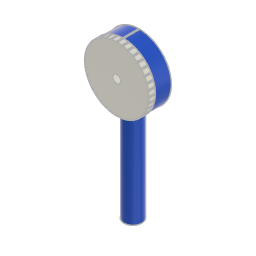
Optica-zelf-geprint (Autodesk Fusion 360 design; units mm, degrees)
Autodesk Fusion 360 part; units mm, degrees
note: some values were not read from the file. Chosen so that the rebuilt part matches the saved one: a side; which face or edge a step refers to. Set by a fixed rule: which sketch regions a step uses.
sketch "Sketch1" plane through (0, 0, 0) normal (0, 1, 0) x (1, 0, 0) in component "Bearing"
  circle A0 centre (0, 0) radius 11
  circle A1 centre (0, 0) radius 4
  dimension "d1" = 22
  dimension "d2" = 8
  constraint coincident A0.centre A1.centre
  measures "d1" diameter of A0
  measures "d2" diameter of A1
extrude "Extrude1" add sketch "Sketch1" along normal blind 7 makes body 1 in component "Bearing"
sketch "Sketch1 (2)" plane through (0, 0, 0) normal (0, -1, 0) x (1, 0, 0) in component "Rotating"
  circle A0 centre (0, 0) radius 4
  circle A1 centre (0, 0) radius 11
  circle A2 centre (0, 0) radius 3.9
  circle A3 centre (0, 0) radius 3.1
  circle A4 centre (0, 0) radius 6.5
  circle A5 centre (0, 0) radius 25
  dimension "d5" = -0.1
  dimension "d10" = -0.9
  dimension "d54" = 2.5
  dimension "d61" = 50
  constraint coincident A0.centre A1.centre
  measures "d61" diameter of A5
extrude "Extrude5" add sketch "Sketch1 (2)" along normal blind 0.5 separate body contours A0 | A4 makes body 2 in component "Rotating"
extrude "Extrude6" add sketch "Sketch1 (2)" along normal up to surface (0.5 mm away) and the other way up to surface (7 mm away) contours A2 bodies 2 in component "Rotating"
extrude "Extrude7" add sketch "Sketch1 (2)" along normal blind 5 from surface at 0.5 contours A0 | A1 | A2 | A4 | A5 bodies 2 in component "Rotating"
sketch "Sketch4" plane through (0, -5.5, 0) normal (0, -1, 0) x (1, 0, 0) in component "Rotating"
  circle A0 centre (0, 0) radius 3.1
  circle A1 centre (0, 0) radius 25
  line L0 (0, 0) -> (0, 25) construction
  line L1 (-0.5, 24.995) -> (0.5, 24.995)
  circle A2 centre (0, 0) radius 25 construction
  line L2 (-0.5, 24.995) -> (0.5, 24.995)
  line L3 (0.5, 24.995) -> (0.5, 24.195)
  line L4 (0.3, 23.995) -> (-0.3, 23.995)
  line L5 (-0.5, 24.195) -> (-0.5, 24.995)
  arc A3 (-0.5, 24.195) -> (-0.3, 23.995) centre (-0.3, 24.195) ccw
  arc A4 (0.3, 23.995) -> (0.5, 24.195) centre (0.3, 24.195) ccw
  line L6 (-3.8479, 24.7021) -> (-3.709, 23.9142)
  arc A5 (-3.8712, 23.6826) -> (-3.709, 23.9142) centre (-3.906, 23.8795) ccw
  line L7 (-3.8712, 23.6826) -> (-4.4621, 23.5784)
  arc A6 (-4.6938, 23.7406) -> (-4.4621, 23.5784) centre (-4.4969, 23.7753) ccw
  line L8 (-4.6938, 23.7406) -> (-4.8327, 24.5284)
  line L9 (-4.8327, 24.5284) -> (-3.8479, 24.7021)
  line L10 (-8.0789, 23.6586) -> (-7.8053, 22.9069)
  arc A7 (-7.9249, 22.6505) -> (-7.8053, 22.9069) centre (-7.9933, 22.8385) ccw
  line L11 (-7.9249, 22.6505) -> (-8.4887, 22.4453)
  arc A8 (-8.745, 22.5649) -> (-8.4887, 22.4453) centre (-8.5571, 22.6333) ccw
  line L12 (-8.745, 22.5649) -> (-9.0186, 23.3166)
  line L13 (-9.0186, 23.3166) -> (-8.0789, 23.6586)
  line L14 (-12.0645, 21.8963) -> (-11.6645, 21.2035)
  arc A9 (-11.7377, 20.9303) -> (-11.6645, 21.2035) centre (-11.8377, 21.1035) ccw
  line L15 (-11.7377, 20.9303) -> (-12.2573, 20.6303)
  arc A10 (-12.5305, 20.7035) -> (-12.2573, 20.6303) centre (-12.3573, 20.8035) ccw
  line L16 (-12.5305, 20.7035) -> (-12.9305, 21.3963)
  line L17 (-12.9305, 21.3963) -> (-12.0645, 21.8963)
  line L18 (-15.6835, 19.4687) -> (-15.1692, 18.8558)
  arc A11 (-15.1939, 18.5741) -> (-15.1692, 18.8558) centre (-15.3224, 18.7273) ccw
  line L19 (-15.1939, 18.5741) -> (-15.6535, 18.1884)
  arc A12 (-15.9353, 18.2131) -> (-15.6535, 18.1884) centre (-15.7821, 18.3416) ccw
  line L20 (-15.9353, 18.2131) -> (-16.4495, 18.8259)
  line L21 (-16.4495, 18.8259) -> (-15.6835, 19.4687)
  line L22 (-18.8259, 16.4495) -> (-18.2131, 15.9353)
  arc A13 (-18.1884, 15.6535) -> (-18.2131, 15.9353) centre (-18.3416, 15.7821) ccw
  line L23 (-18.1884, 15.6535) -> (-18.5741, 15.1939)
  arc A14 (-18.8558, 15.1692) -> (-18.5741, 15.1939) centre (-18.7273, 15.3224) ccw
  line L24 (-18.8558, 15.1692) -> (-19.4687, 15.6835)
  line L25 (-19.4687, 15.6835) -> (-18.8259, 16.4495)
  line L26 (-21.3963, 12.9305) -> (-20.7035, 12.5305)
  arc A15 (-20.6303, 12.2573) -> (-20.7035, 12.5305) centre (-20.8035, 12.3573) ccw
  line L27 (-20.6303, 12.2573) -> (-20.9303, 11.7377)
  arc A16 (-21.2035, 11.6645) -> (-20.9303, 11.7377) centre (-21.1035, 11.8377) ccw
  line L28 (-21.2035, 11.6645) -> (-21.8963, 12.0645)
  line L29 (-21.8963, 12.0645) -> (-21.3963, 12.9305)
  line L30 (-23.3166, 9.0186) -> (-22.5649, 8.745)
  arc A17 (-22.4453, 8.4887) -> (-22.5649, 8.745) centre (-22.6333, 8.5571) ccw
  line L31 (-22.4453, 8.4887) -> (-22.6505, 7.9249)
  arc A18 (-22.9069, 7.8053) -> (-22.6505, 7.9249) centre (-22.8385, 7.9933) ccw
  line L32 (-22.9069, 7.8053) -> (-23.6586, 8.0789)
  line L33 (-23.6586, 8.0789) -> (-23.3166, 9.0186)
  line L34 (-24.5284, 4.8327) -> (-23.7406, 4.6938)
  arc A19 (-23.5784, 4.4621) -> (-23.7406, 4.6938) centre (-23.7753, 4.4969) ccw
  line L35 (-23.5784, 4.4621) -> (-23.6826, 3.8712)
  arc A20 (-23.9142, 3.709) -> (-23.6826, 3.8712) centre (-23.8795, 3.906) ccw
  line L36 (-23.9142, 3.709) -> (-24.7021, 3.8479)
  line L37 (-24.7021, 3.8479) -> (-24.5284, 4.8327)
  line L38 (-24.995, 0.5) -> (-24.195, 0.5)
  arc A21 (-23.995, 0.3) -> (-24.195, 0.5) centre (-24.195, 0.3) ccw
  line L39 (-23.995, 0.3) -> (-23.995, -0.3)
  arc A22 (-24.195, -0.5) -> (-23.995, -0.3) centre (-24.195, -0.3) ccw
  line L40 (-24.195, -0.5) -> (-24.995, -0.5)
  line L41 (-24.995, -0.5) -> (-24.995, 0.5)
  line L42 (-24.7021, -3.8479) -> (-23.9142, -3.709)
  arc A23 (-23.6826, -3.8712) -> (-23.9142, -3.709) centre (-23.8795, -3.906) ccw
  line L43 (-23.6826, -3.8712) -> (-23.5784, -4.4621)
  arc A24 (-23.7406, -4.6938) -> (-23.5784, -4.4621) centre (-23.7753, -4.4969) ccw
  line L44 (-23.7406, -4.6938) -> (-24.5284, -4.8327)
  line L45 (-24.5284, -4.8327) -> (-24.7021, -3.8479)
  line L46 (-23.6586, -8.0789) -> (-22.9069, -7.8053)
  arc A25 (-22.6505, -7.9249) -> (-22.9069, -7.8053) centre (-22.8385, -7.9933) ccw
  line L47 (-22.6505, -7.9249) -> (-22.4453, -8.4887)
  arc A26 (-22.5649, -8.745) -> (-22.4453, -8.4887) centre (-22.6333, -8.5571) ccw
  line L48 (-22.5649, -8.745) -> (-23.3166, -9.0186)
  line L49 (-23.3166, -9.0186) -> (-23.6586, -8.0789)
  line L50 (-21.8963, -12.0645) -> (-21.2035, -11.6645)
  arc A27 (-20.9303, -11.7377) -> (-21.2035, -11.6645) centre (-21.1035, -11.8377) ccw
  line L51 (-20.9303, -11.7377) -> (-20.6303, -12.2573)
  arc A28 (-20.7035, -12.5305) -> (-20.6303, -12.2573) centre (-20.8035, -12.3573) ccw
  line L52 (-20.7035, -12.5305) -> (-21.3963, -12.9305)
  line L53 (-21.3963, -12.9305) -> (-21.8963, -12.0645)
  line L54 (-19.4687, -15.6835) -> (-18.8558, -15.1692)
  arc A29 (-18.5741, -15.1939) -> (-18.8558, -15.1692) centre (-18.7273, -15.3224) ccw
  line L55 (-18.5741, -15.1939) -> (-18.1884, -15.6535)
  arc A30 (-18.2131, -15.9353) -> (-18.1884, -15.6535) centre (-18.3416, -15.7821) ccw
  line L56 (-18.2131, -15.9353) -> (-18.8259, -16.4495)
  line L57 (-18.8259, -16.4495) -> (-19.4687, -15.6835)
  line L58 (-16.4495, -18.8259) -> (-15.9353, -18.2131)
  arc A31 (-15.6535, -18.1884) -> (-15.9353, -18.2131) centre (-15.7821, -18.3416) ccw
  line L59 (-15.6535, -18.1884) -> (-15.1939, -18.5741)
  arc A32 (-15.1692, -18.8558) -> (-15.1939, -18.5741) centre (-15.3224, -18.7273) ccw
  line L60 (-15.1692, -18.8558) -> (-15.6835, -19.4687)
  line L61 (-15.6835, -19.4687) -> (-16.4495, -18.8259)
  line L62 (-12.9305, -21.3963) -> (-12.5305, -20.7035)
  arc A33 (-12.2573, -20.6303) -> (-12.5305, -20.7035) centre (-12.3573, -20.8035) ccw
  line L63 (-12.2573, -20.6303) -> (-11.7377, -20.9303)
  arc A34 (-11.6645, -21.2035) -> (-11.7377, -20.9303) centre (-11.8377, -21.1035) ccw
  line L64 (-11.6645, -21.2035) -> (-12.0645, -21.8963)
  line L65 (-12.0645, -21.8963) -> (-12.9305, -21.3963)
  line L66 (-9.0186, -23.3166) -> (-8.745, -22.5649)
  arc A35 (-8.4887, -22.4453) -> (-8.745, -22.5649) centre (-8.5571, -22.6333) ccw
  line L67 (-8.4887, -22.4453) -> (-7.9249, -22.6505)
  arc A36 (-7.8053, -22.9069) -> (-7.9249, -22.6505) centre (-7.9933, -22.8385) ccw
  line L68 (-7.8053, -22.9069) -> (-8.0789, -23.6586)
  line L69 (-8.0789, -23.6586) -> (-9.0186, -23.3166)
  line L70 (-4.8327, -24.5284) -> (-4.6938, -23.7406)
  arc A37 (-4.4621, -23.5784) -> (-4.6938, -23.7406) centre (-4.4969, -23.7753) ccw
  line L71 (-4.4621, -23.5784) -> (-3.8712, -23.6826)
  arc A38 (-3.709, -23.9142) -> (-3.8712, -23.6826) centre (-3.906, -23.8795) ccw
  line L72 (-3.709, -23.9142) -> (-3.8479, -24.7021)
  line L73 (-3.8479, -24.7021) -> (-4.8327, -24.5284)
  line L74 (-0.5, -24.995) -> (-0.5, -24.195)
  arc A39 (-0.3, -23.995) -> (-0.5, -24.195) centre (-0.3, -24.195) ccw
  line L75 (-0.3, -23.995) -> (0.3, -23.995)
  arc A40 (0.5, -24.195) -> (0.3, -23.995) centre (0.3, -24.195) ccw
  line L76 (0.5, -24.195) -> (0.5, -24.995)
  line L77 (0.5, -24.995) -> (-0.5, -24.995)
  line L78 (3.8479, -24.7021) -> (3.709, -23.9142)
  arc A41 (3.8712, -23.6826) -> (3.709, -23.9142) centre (3.906, -23.8795) ccw
  line L79 (3.8712, -23.6826) -> (4.4621, -23.5784)
  arc A42 (4.6938, -23.7406) -> (4.4621, -23.5784) centre (4.4969, -23.7753) ccw
  line L80 (4.6938, -23.7406) -> (4.8327, -24.5284)
  line L81 (4.8327, -24.5284) -> (3.8479, -24.7021)
  line L82 (8.0789, -23.6586) -> (7.8053, -22.9069)
  arc A43 (7.9249, -22.6505) -> (7.8053, -22.9069) centre (7.9933, -22.8385) ccw
  line L83 (7.9249, -22.6505) -> (8.4887, -22.4453)
  arc A44 (8.745, -22.5649) -> (8.4887, -22.4453) centre (8.5571, -22.6333) ccw
  line L84 (8.745, -22.5649) -> (9.0186, -23.3166)
  line L85 (9.0186, -23.3166) -> (8.0789, -23.6586)
  line L86 (12.0645, -21.8963) -> (11.6645, -21.2035)
  arc A45 (11.7377, -20.9303) -> (11.6645, -21.2035) centre (11.8377, -21.1035) ccw
  line L87 (11.7377, -20.9303) -> (12.2573, -20.6303)
  arc A46 (12.5305, -20.7035) -> (12.2573, -20.6303) centre (12.3573, -20.8035) ccw
  line L88 (12.5305, -20.7035) -> (12.9305, -21.3963)
  line L89 (12.9305, -21.3963) -> (12.0645, -21.8963)
  line L90 (15.6835, -19.4687) -> (15.1692, -18.8558)
  arc A47 (15.1939, -18.5741) -> (15.1692, -18.8558) centre (15.3224, -18.7273) ccw
  line L91 (15.1939, -18.5741) -> (15.6535, -18.1884)
  arc A48 (15.9353, -18.2131) -> (15.6535, -18.1884) centre (15.7821, -18.3416) ccw
  line L92 (15.9353, -18.2131) -> (16.4495, -18.8259)
  line L93 (16.4495, -18.8259) -> (15.6835, -19.4687)
  line L94 (18.8259, -16.4495) -> (18.2131, -15.9353)
  arc A49 (18.1884, -15.6535) -> (18.2131, -15.9353) centre (18.3416, -15.7821) ccw
  line L95 (18.1884, -15.6535) -> (18.5741, -15.1939)
  arc A50 (18.8558, -15.1692) -> (18.5741, -15.1939) centre (18.7273, -15.3224) ccw
  line L96 (18.8558, -15.1692) -> (19.4687, -15.6835)
  line L97 (19.4687, -15.6835) -> (18.8259, -16.4495)
  line L98 (21.3963, -12.9305) -> (20.7035, -12.5305)
  arc A51 (20.6303, -12.2573) -> (20.7035, -12.5305) centre (20.8035, -12.3573) ccw
  line L99 (20.6303, -12.2573) -> (20.9303, -11.7377)
  arc A52 (21.2035, -11.6645) -> (20.9303, -11.7377) centre (21.1035, -11.8377) ccw
  line L100 (21.2035, -11.6645) -> (21.8963, -12.0645)
  line L101 (21.8963, -12.0645) -> (21.3963, -12.9305)
  line L102 (23.3166, -9.0186) -> (22.5649, -8.745)
  arc A53 (22.4453, -8.4887) -> (22.5649, -8.745) centre (22.6333, -8.5571) ccw
  line L103 (22.4453, -8.4887) -> (22.6505, -7.9249)
  arc A54 (22.9069, -7.8053) -> (22.6505, -7.9249) centre (22.8385, -7.9933) ccw
  line L104 (22.9069, -7.8053) -> (23.6586, -8.0789)
  line L105 (23.6586, -8.0789) -> (23.3166, -9.0186)
  line L106 (24.5284, -4.8327) -> (23.7406, -4.6938)
  arc A55 (23.5784, -4.4621) -> (23.7406, -4.6938) centre (23.7753, -4.4969) ccw
  line L107 (23.5784, -4.4621) -> (23.6826, -3.8712)
  arc A56 (23.9142, -3.709) -> (23.6826, -3.8712) centre (23.8795, -3.906) ccw
  line L108 (23.9142, -3.709) -> (24.7021, -3.8479)
  line L109 (24.7021, -3.8479) -> (24.5284, -4.8327)
  line L110 (24.995, -0.5) -> (24.195, -0.5)
  arc A57 (23.995, -0.3) -> (24.195, -0.5) centre (24.195, -0.3) ccw
  line L111 (23.995, -0.3) -> (23.995, 0.3)
  arc A58 (24.195, 0.5) -> (23.995, 0.3) centre (24.195, 0.3) ccw
  line L112 (24.195, 0.5) -> (24.995, 0.5)
  line L113 (24.995, 0.5) -> (24.995, -0.5)
  line L114 (24.7021, 3.8479) -> (23.9142, 3.709)
  arc A59 (23.6826, 3.8712) -> (23.9142, 3.709) centre (23.8795, 3.906) ccw
  line L115 (23.6826, 3.8712) -> (23.5784, 4.4621)
  arc A60 (23.7406, 4.6938) -> (23.5784, 4.4621) centre (23.7753, 4.4969) ccw
  line L116 (23.7406, 4.6938) -> (24.5284, 4.8327)
  line L117 (24.5284, 4.8327) -> (24.7021, 3.8479)
  line L118 (23.6586, 8.0789) -> (22.9069, 7.8053)
  arc A61 (22.6505, 7.9249) -> (22.9069, 7.8053) centre (22.8385, 7.9933) ccw
  line L119 (22.6505, 7.9249) -> (22.4453, 8.4887)
  arc A62 (22.5649, 8.745) -> (22.4453, 8.4887) centre (22.6333, 8.5571) ccw
  line L120 (22.5649, 8.745) -> (23.3166, 9.0186)
  line L121 (23.3166, 9.0186) -> (23.6586, 8.0789)
  line L122 (21.8963, 12.0645) -> (21.2035, 11.6645)
  arc A63 (20.9303, 11.7377) -> (21.2035, 11.6645) centre (21.1035, 11.8377) ccw
  line L123 (20.9303, 11.7377) -> (20.6303, 12.2573)
  arc A64 (20.7035, 12.5305) -> (20.6303, 12.2573) centre (20.8035, 12.3573) ccw
  line L124 (20.7035, 12.5305) -> (21.3963, 12.9305)
  line L125 (21.3963, 12.9305) -> (21.8963, 12.0645)
  line L126 (19.4687, 15.6835) -> (18.8558, 15.1692)
  arc A65 (18.5741, 15.1939) -> (18.8558, 15.1692) centre (18.7273, 15.3224) ccw
  line L127 (18.5741, 15.1939) -> (18.1884, 15.6535)
  arc A66 (18.2131, 15.9353) -> (18.1884, 15.6535) centre (18.3416, 15.7821) ccw
  line L128 (18.2131, 15.9353) -> (18.8259, 16.4495)
  line L129 (18.8259, 16.4495) -> (19.4687, 15.6835)
  line L130 (16.4495, 18.8259) -> (15.9353, 18.2131)
  arc A67 (15.6535, 18.1884) -> (15.9353, 18.2131) centre (15.7821, 18.3416) ccw
  line L131 (15.6535, 18.1884) -> (15.1939, 18.5741)
  arc A68 (15.1692, 18.8558) -> (15.1939, 18.5741) centre (15.3224, 18.7273) ccw
  line L132 (15.1692, 18.8558) -> (15.6835, 19.4687)
  line L133 (15.6835, 19.4687) -> (16.4495, 18.8259)
  line L134 (12.9305, 21.3963) -> (12.5305, 20.7035)
  arc A69 (12.2573, 20.6303) -> (12.5305, 20.7035) centre (12.3573, 20.8035) ccw
  line L135 (12.2573, 20.6303) -> (11.7377, 20.9303)
  arc A70 (11.6645, 21.2035) -> (11.7377, 20.9303) centre (11.8377, 21.1035) ccw
  line L136 (11.6645, 21.2035) -> (12.0645, 21.8963)
  line L137 (12.0645, 21.8963) -> (12.9305, 21.3963)
  line L138 (9.0186, 23.3166) -> (8.745, 22.5649)
  arc A71 (8.4887, 22.4453) -> (8.745, 22.5649) centre (8.5571, 22.6333) ccw
  line L139 (8.4887, 22.4453) -> (7.9249, 22.6505)
  arc A72 (7.8053, 22.9069) -> (7.9249, 22.6505) centre (7.9933, 22.8385) ccw
  line L140 (7.8053, 22.9069) -> (8.0789, 23.6586)
  line L141 (8.0789, 23.6586) -> (9.0186, 23.3166)
  line L142 (4.8327, 24.5284) -> (4.6938, 23.7406)
  arc A73 (4.4621, 23.5784) -> (4.6938, 23.7406) centre (4.4969, 23.7753) ccw
  line L143 (4.4621, 23.5784) -> (3.8712, 23.6826)
  arc A74 (3.709, 23.9142) -> (3.8712, 23.6826) centre (3.906, 23.8795) ccw
  line L144 (3.709, 23.9142) -> (3.8479, 24.7021)
  line L145 (3.8479, 24.7021) -> (4.8327, 24.5284)
  line L146 (-4.7516, 24.6443) -> (-3.9638, 24.7832)
  line L147 (-3.8479, 24.7021) -> (-4.8327, 24.5284)
  arc A75 (-4.7516, 24.6443) -> (-4.8327, 24.5284) centre (-4.7343, 24.5458) ccw
  arc A76 (-3.8479, 24.7021) -> (-3.9638, 24.7832) centre (-3.9464, 24.6847) ccw
  point P0 (0, 24.995)
  point P1 (-0.5, 23.995)
  dimension "d65" = 1
  dimension "d70" = 1
  dimension "d71" = 0.2
  dimension "d73" = 360
  dimension "d76" = 0.1
  dimension "d77" = 0.1
  dimension "d78" = 0.8
  constraint coincident A0.centre A1.centre
  constraint coincident A1 L0.end
  constraint vertical L0
  constraint perpendicular L0 L1
  constraint midpoint L1 P0
  constraint coincident L0 P0
  constraint coincident L1.start A2
  constraint perpendicular L2 L3
  constraint parallel L2 L4
  constraint parallel L3 L5
  constraint coincident P1 L4
  constraint coincident P1 L5
  constraint tangent L4 A3
  constraint tangent L5 A3
  constraint tangent L3 A4
  constraint tangent L4 A4
  constraint equal A3 A4
  constraint parallel L146 L147
  constraint tangent L146 A75
  constraint coincident L8.end L9.start
  constraint tangent L146 A76
  constraint equal A75 A76
  constraint coincident L6.start L9.end
  measures "d65" distance of L1.start L1.end
  measures "d70" distance of L1.start P1
  measures "d71" radius of A3
  measures "d76" radius of A75
  measures "d77" distance of L146 L147
  measures "d78" distance of L146.start L146.end
extrude "Extrude8" add sketch "Sketch4" against normal blind 5 contours A1 L146 A75 A76 bodies 2 in component "Rotating"
pattern_circular "C-Pattern1" count 36 over 360 about axis through (0, 1.75, 0) along (0, 1, 0) of "Extrude8" in component "Rotating"
extrude "Extrude9" cut sketch "Sketch4" against normal blind 0.001 contours L110 A57 L111 A58 L112 L113 | L114 A59 L115 A60 L116 L117 | L106 A55 L107 A56 L108 L109 | L118 A61 L119 A62 L120 L121 | L102 A53 L103 A54 L104 L105 | L122 A63 L123 A64 L124 L125 | L98 A51 L99 A52 L100 L101 | L126 A65 L127 A66 L128 L129 | L94 A49 L95 A50 L96 L97 | L130 A67 L131 A68 L132 L133 | L90 A47 L91 A48 L92 L93 | L134 A69 L135 A70 L136 L137 | L86 A45 L87 A46 L88 L89 | L138 A71 L139 A72 L140 L141 | L82 A43 L83 A44 L84 L85 | L142 A73 L143 A74 L144 L145 | L78 A41 L79 A42 L80 L81 | L1 L2 L3 L4 L5 A3 A4 | L74 A39 L75 A40 L76 L77 | L6 A5 L7 A6 L8 L9 L147 | L70 A37 L71 A38 L72 L73 | L10 A7 L11 A8 L12 L13 | L66 A35 L67 A36 L68 L69 | L14 A9 L15 A10 L16 L17 | L62 A33 L63 A34 L64 L65 | L18 A11 L19 A12 L20 L21 | L58 A31 L59 A32 L60 L61 | L22 A13 L23 A14 L24 L25 | L54 A29 L55 A30 L56 L57 | L26 A15 L27 A16 L28 L29 | L50 A27 L51 A28 L52 L53 | L30 A17 L31 A18 L32 L33 | L46 A25 L47 A26 L48 L49 | L34 A19 L35 A20 L36 L37 | L42 A23 L43 A24 L44 L45 | L38 A21 L39 A22 L40 L41 bodies 2 in component "Rotating"
sketch "Sketch1 (3)" plane through (0, 7, 0) normal (0, 1, 0) x (-1, 0, 0) in component "Static"
  circle A0 centre (0, 0) radius 4
  circle A1 centre (0, 0) radius 11
  circle A2 centre (0, 0) radius 3.1
  circle A3 centre (0, 0) radius 3.9
  arc A4 (3.8479, 24.7021) -> (0.5, 24.995) centre (0, 0) ccw
  arc A5 (0.5, 24.995) -> (0.4, 25.095) centre (0.4, 24.995) ccw
  line L0 (0.4, 25.095) -> (-0.4, 25.095)
  arc A6 (-0.4, 25.095) -> (-0.5, 24.995) centre (-0.4, 24.995) ccw
  arc A7 (-0.5, 24.995) -> (-3.8479, 24.7021) centre (0, 0) ccw
  arc A8 (-3.8479, 24.7021) -> (-3.9638, 24.7832) centre (-3.9464, 24.6847) ccw
  line L1 (-3.9638, 24.7832) -> (-4.7516, 24.6443)
  arc A9 (-4.7516, 24.6443) -> (-4.8327, 24.5284) centre (-4.7343, 24.5458) ccw
  arc A10 (-4.8327, 24.5284) -> (-8.0789, 23.6586) centre (0, 0) ccw
  arc A11 (-8.0789, 23.6586) -> (-8.2071, 23.7184) centre (-8.1729, 23.6244) ccw
  line L2 (-8.2071, 23.7184) -> (-8.9589, 23.4448)
  arc A12 (-8.9589, 23.4448) -> (-9.0186, 23.3166) centre (-8.9247, 23.3508) ccw
  arc A13 (-9.0186, 23.3166) -> (-12.0645, 21.8963) centre (0, 0) ccw
  arc A14 (-12.0645, 21.8963) -> (-12.2011, 21.9329) centre (-12.1511, 21.8463) ccw
  line L3 (-12.2011, 21.9329) -> (-12.8939, 21.5329)
  arc A15 (-12.8939, 21.5329) -> (-12.9305, 21.3963) centre (-12.8439, 21.4463) ccw
  arc A16 (-12.9305, 21.3963) -> (-15.6835, 19.4687) centre (0, 0) ccw
  arc A17 (-15.6835, 19.4687) -> (-15.8243, 19.481) centre (-15.7601, 19.4044) ccw
  line L4 (-15.8243, 19.481) -> (-16.4372, 18.9668)
  arc A18 (-16.4372, 18.9668) -> (-16.4495, 18.8259) centre (-16.3729, 18.8902) ccw
  arc A19 (-16.4495, 18.8259) -> (-18.8259, 16.4495) centre (0, 0) ccw
  arc A20 (-18.8259, 16.4495) -> (-18.9668, 16.4372) centre (-18.8902, 16.3729) ccw
  line L5 (-18.9668, 16.4372) -> (-19.481, 15.8243)
  arc A21 (-19.481, 15.8243) -> (-19.4687, 15.6835) centre (-19.4044, 15.7601) ccw
  arc A22 (-19.4687, 15.6835) -> (-21.3963, 12.9305) centre (0, 0) ccw
  arc A23 (-21.3963, 12.9305) -> (-21.5329, 12.8939) centre (-21.4463, 12.8439) ccw
  line L6 (-21.5329, 12.8939) -> (-21.9329, 12.2011)
  arc A24 (-21.9329, 12.2011) -> (-21.8963, 12.0645) centre (-21.8463, 12.1511) ccw
  arc A25 (-21.8963, 12.0645) -> (-23.3166, 9.0186) centre (0, 0) ccw
  arc A26 (-23.3166, 9.0186) -> (-23.4448, 8.9589) centre (-23.3508, 8.9247) ccw
  line L7 (-23.4448, 8.9589) -> (-23.7184, 8.2071)
  arc A27 (-23.7184, 8.2071) -> (-23.6586, 8.0789) centre (-23.6244, 8.1729) ccw
  arc A28 (-23.6586, 8.0789) -> (-24.5284, 4.8327) centre (0, 0) ccw
  arc A29 (-24.5284, 4.8327) -> (-24.6443, 4.7516) centre (-24.5458, 4.7343) ccw
  line L8 (-24.6443, 4.7516) -> (-24.7832, 3.9638)
  arc A30 (-24.7832, 3.9638) -> (-24.7021, 3.8479) centre (-24.6847, 3.9464) ccw
  arc A31 (-24.7021, 3.8479) -> (-24.995, 0.5) centre (0, 0) ccw
  arc A32 (-24.995, 0.5) -> (-25.095, 0.4) centre (-24.995, 0.4) ccw
  line L9 (-25.095, 0.4) -> (-25.095, -0.4)
  arc A33 (-25.095, -0.4) -> (-24.995, -0.5) centre (-24.995, -0.4) ccw
  arc A34 (-24.995, -0.5) -> (-24.7021, -3.8479) centre (0, 0) ccw
  arc A35 (-24.7021, -3.8479) -> (-24.7832, -3.9638) centre (-24.6847, -3.9464) ccw
  line L10 (-24.7832, -3.9638) -> (-24.6443, -4.7516)
  arc A36 (-24.6443, -4.7516) -> (-24.5284, -4.8327) centre (-24.5458, -4.7343) ccw
  arc A37 (-24.5284, -4.8327) -> (-23.6586, -8.0789) centre (0, 0) ccw
  arc A38 (-23.6586, -8.0789) -> (-23.7184, -8.2071) centre (-23.6244, -8.1729) ccw
  line L11 (-23.7184, -8.2071) -> (-23.4448, -8.9589)
  arc A39 (-23.4448, -8.9589) -> (-23.3166, -9.0186) centre (-23.3508, -8.9247) ccw
  arc A40 (-23.3166, -9.0186) -> (-21.8963, -12.0645) centre (0, 0) ccw
  arc A41 (-21.8963, -12.0645) -> (-21.9329, -12.2011) centre (-21.8463, -12.1511) ccw
  line L12 (-21.9329, -12.2011) -> (-21.5329, -12.8939)
  arc A42 (-21.5329, -12.8939) -> (-21.3963, -12.9305) centre (-21.4463, -12.8439) ccw
  arc A43 (-21.3963, -12.9305) -> (-19.4687, -15.6835) centre (0, 0) ccw
  arc A44 (-19.4687, -15.6835) -> (-19.481, -15.8243) centre (-19.4044, -15.7601) ccw
  line L13 (-19.481, -15.8243) -> (-18.9668, -16.4372)
  arc A45 (-18.9668, -16.4372) -> (-18.8259, -16.4495) centre (-18.8902, -16.3729) ccw
  arc A46 (-18.8259, -16.4495) -> (-16.4495, -18.8259) centre (0, 0) ccw
  arc A47 (-16.4495, -18.8259) -> (-16.4372, -18.9668) centre (-16.3729, -18.8902) ccw
  line L14 (-16.4372, -18.9668) -> (-15.8243, -19.481)
  arc A48 (-15.8243, -19.481) -> (-15.6835, -19.4687) centre (-15.7601, -19.4044) ccw
  arc A49 (-15.6835, -19.4687) -> (-12.9305, -21.3963) centre (0, 0) ccw
  arc A50 (-12.9305, -21.3963) -> (-12.8939, -21.5329) centre (-12.8439, -21.4463) ccw
  line L15 (-12.8939, -21.5329) -> (-12.2011, -21.9329)
  arc A51 (-12.2011, -21.9329) -> (-12.0645, -21.8963) centre (-12.1511, -21.8463) ccw
  arc A52 (-12.0645, -21.8963) -> (-9.0186, -23.3166) centre (0, 0) ccw
  arc A53 (-9.0186, -23.3166) -> (-8.9589, -23.4448) centre (-8.9247, -23.3508) ccw
  line L16 (-8.9589, -23.4448) -> (-8.2071, -23.7184)
  arc A54 (-8.2071, -23.7184) -> (-8.0789, -23.6586) centre (-8.1729, -23.6244) ccw
  arc A55 (-8.0789, -23.6586) -> (-4.8327, -24.5284) centre (0, 0) ccw
  arc A56 (-4.8327, -24.5284) -> (-4.7516, -24.6443) centre (-4.7343, -24.5458) ccw
  line L17 (-4.7516, -24.6443) -> (-3.9638, -24.7832)
  arc A57 (-3.9638, -24.7832) -> (-3.8479, -24.7021) centre (-3.9464, -24.6847) ccw
  arc A58 (-3.8479, -24.7021) -> (-0.5, -24.995) centre (0, 0) ccw
  arc A59 (-0.5, -24.995) -> (-0.4, -25.095) centre (-0.4, -24.995) ccw
  line L18 (-0.4, -25.095) -> (0.4, -25.095)
  arc A60 (0.4, -25.095) -> (0.5, -24.995) centre (0.4, -24.995) ccw
  arc A61 (0.5, -24.995) -> (3.8479, -24.7021) centre (0, 0) ccw
  arc A62 (3.8479, -24.7021) -> (3.9638, -24.7832) centre (3.9464, -24.6847) ccw
  line L19 (3.9638, -24.7832) -> (4.7516, -24.6443)
  arc A63 (4.7516, -24.6443) -> (4.8327, -24.5284) centre (4.7343, -24.5458) ccw
  arc A64 (4.8327, -24.5284) -> (8.0789, -23.6586) centre (0, 0) ccw
  arc A65 (8.0789, -23.6586) -> (8.2071, -23.7184) centre (8.1729, -23.6244) ccw
  line L20 (8.2071, -23.7184) -> (8.9589, -23.4448)
  arc A66 (8.9589, -23.4448) -> (9.0186, -23.3166) centre (8.9247, -23.3508) ccw
  arc A67 (9.0186, -23.3166) -> (12.0645, -21.8963) centre (0, 0) ccw
  arc A68 (12.0645, -21.8963) -> (12.2011, -21.9329) centre (12.1511, -21.8463) ccw
  line L21 (12.2011, -21.9329) -> (12.8939, -21.5329)
  arc A69 (12.8939, -21.5329) -> (12.9305, -21.3963) centre (12.8439, -21.4463) ccw
  arc A70 (12.9305, -21.3963) -> (15.6835, -19.4687) centre (0, 0) ccw
  arc A71 (15.6835, -19.4687) -> (15.8243, -19.481) centre (15.7601, -19.4044) ccw
  line L22 (15.8243, -19.481) -> (16.4372, -18.9668)
  arc A72 (16.4372, -18.9668) -> (16.4495, -18.8259) centre (16.3729, -18.8902) ccw
  arc A73 (16.4495, -18.8259) -> (18.8259, -16.4495) centre (0, 0) ccw
  arc A74 (18.8259, -16.4495) -> (18.9668, -16.4372) centre (18.8902, -16.3729) ccw
  line L23 (18.9668, -16.4372) -> (19.481, -15.8243)
  arc A75 (19.481, -15.8243) -> (19.4687, -15.6835) centre (19.4044, -15.7601) ccw
  arc A76 (19.4687, -15.6835) -> (21.3963, -12.9305) centre (0, 0) ccw
  arc A77 (21.3963, -12.9305) -> (21.5329, -12.8939) centre (21.4463, -12.8439) ccw
  line L24 (21.5329, -12.8939) -> (21.9329, -12.2011)
  arc A78 (21.9329, -12.2011) -> (21.8963, -12.0645) centre (21.8463, -12.1511) ccw
  arc A79 (21.8963, -12.0645) -> (23.3166, -9.0186) centre (0, 0) ccw
  arc A80 (23.3166, -9.0186) -> (23.4448, -8.9589) centre (23.3508, -8.9247) ccw
  line L25 (23.4448, -8.9589) -> (23.7184, -8.2071)
  arc A81 (23.7184, -8.2071) -> (23.6586, -8.0789) centre (23.6244, -8.1729) ccw
  arc A82 (23.6586, -8.0789) -> (24.5284, -4.8327) centre (0, 0) ccw
  arc A83 (24.5284, -4.8327) -> (24.6443, -4.7516) centre (24.5458, -4.7343) ccw
  line L26 (24.6443, -4.7516) -> (24.7832, -3.9638)
  arc A84 (24.7832, -3.9638) -> (24.7021, -3.8479) centre (24.6847, -3.9464) ccw
  arc A85 (24.7021, -3.8479) -> (24.995, -0.5) centre (0, 0) ccw
  arc A86 (24.995, -0.5) -> (25.095, -0.4) centre (24.995, -0.4) ccw
  line L27 (25.095, -0.4) -> (25.095, 0.4)
  arc A87 (25.095, 0.4) -> (24.995, 0.5) centre (24.995, 0.4) ccw
  arc A88 (24.995, 0.5) -> (24.7021, 3.8479) centre (0, 0) ccw
  arc A89 (24.7021, 3.8479) -> (24.7832, 3.9638) centre (24.6847, 3.9464) ccw
  line L28 (24.7832, 3.9638) -> (24.6443, 4.7516)
  arc A90 (24.6443, 4.7516) -> (24.5284, 4.8327) centre (24.5458, 4.7343) ccw
  arc A91 (24.5284, 4.8327) -> (23.6586, 8.0789) centre (0, 0) ccw
  arc A92 (23.6586, 8.0789) -> (23.7184, 8.2071) centre (23.6244, 8.1729) ccw
  line L29 (23.7184, 8.2071) -> (23.4448, 8.9589)
  arc A93 (23.4448, 8.9589) -> (23.3166, 9.0186) centre (23.3508, 8.9247) ccw
  arc A94 (23.3166, 9.0186) -> (21.8963, 12.0645) centre (0, 0) ccw
  arc A95 (21.8963, 12.0645) -> (21.9329, 12.2011) centre (21.8463, 12.1511) ccw
  line L30 (21.9329, 12.2011) -> (21.5329, 12.8939)
  arc A96 (21.5329, 12.8939) -> (21.3963, 12.9305) centre (21.4463, 12.8439) ccw
  arc A97 (21.3963, 12.9305) -> (19.4687, 15.6835) centre (0, 0) ccw
  arc A98 (19.4687, 15.6835) -> (19.481, 15.8243) centre (19.4044, 15.7601) ccw
  line L31 (19.481, 15.8243) -> (18.9668, 16.4372)
  arc A99 (18.9668, 16.4372) -> (18.8259, 16.4495) centre (18.8902, 16.3729) ccw
  arc A100 (18.8259, 16.4495) -> (16.4495, 18.8259) centre (0, 0) ccw
  arc A101 (16.4495, 18.8259) -> (16.4372, 18.9668) centre (16.3729, 18.8902) ccw
  line L32 (16.4372, 18.9668) -> (15.8243, 19.481)
  arc A102 (15.8243, 19.481) -> (15.6835, 19.4687) centre (15.7601, 19.4044) ccw
  arc A103 (15.6835, 19.4687) -> (12.9305, 21.3963) centre (0, 0) ccw
  arc A104 (12.9305, 21.3963) -> (12.8939, 21.5329) centre (12.8439, 21.4463) ccw
  line L33 (12.8939, 21.5329) -> (12.2011, 21.9329)
  arc A105 (12.2011, 21.9329) -> (12.0645, 21.8963) centre (12.1511, 21.8463) ccw
  arc A106 (12.0645, 21.8963) -> (9.0186, 23.3166) centre (0, 0) ccw
  arc A107 (9.0186, 23.3166) -> (8.9589, 23.4448) centre (8.9247, 23.3508) ccw
  line L34 (8.9589, 23.4448) -> (8.2071, 23.7184)
  arc A108 (8.2071, 23.7184) -> (8.0789, 23.6586) centre (8.1729, 23.6244) ccw
  arc A109 (8.0789, 23.6586) -> (4.8327, 24.5284) centre (0, 0) ccw
  arc A110 (4.8327, 24.5284) -> (4.7516, 24.6443) centre (4.7343, 24.5458) ccw
  line L35 (4.7516, 24.6443) -> (3.9638, 24.7832)
  arc A111 (3.9638, 24.7832) -> (3.8479, 24.7021) centre (3.9464, 24.6847) ccw
  circle A112 centre (0, 0) radius 6.5
  circle A113 centre (0, 0) radius 11.1
  circle A114 centre (0, 0) radius 25
  dimension "d79" = 0.1
  dimension "d80" = 50
  constraint concentric A4 A114
  measures "d80" diameter of A114
extrude "Extrude1'" add sketch "Sketch1 (3)" against normal up to surface (12.4 mm away) from surface at 5 separate body contours A4 A7 A10 A13 A16 A19 A22 A25 A28 A31 A34 A37 A40 A43 A46 A49 A52 A55 A58 A61 A64 A67 A70 A73 A76 A79 A82 A85 A88 A91 A94 A97 A100 A103 A106 A109 A114 | A5 L0 A6 A114 | A86 L27 A87 A114 makes body 3 in component "Static"
sketch "Sketch6" plane through (0, 12, 0) normal (0, 1, 0) x (-1, 0, 0) in component "Static"
  circle A0 centre (0, 0) radius 11.1
  arc A1 (25.095, 0.4) -> (24.995, 0.5) centre (24.995, 0.4) ccw
  arc A2 (24.995, 0.5) -> (0.5, 24.995) centre (0, 0) ccw
  arc A3 (0.5, 24.995) -> (0.4, 25.095) centre (0.4, 24.995) ccw
  line L0 (0.4, 25.095) -> (-0.4, 25.095)
  arc A4 (-0.4, 25.095) -> (-0.5, 24.995) centre (-0.4, 24.995) ccw
  arc A5 (-0.5, 24.995) -> (24.995, -0.5) centre (0, 0) ccw
  arc A6 (24.995, -0.5) -> (25.095, -0.4) centre (24.995, -0.4) ccw
  line L1 (25.095, -0.4) -> (25.095, 0.4)
  circle A7 centre (0, 0) radius 4
extrude "Extrude3" add sketch "Sketch6" against normal up to surface (4.5 mm away) contours A0 bodies 3 in component "Static"
sketch "Sketch7" plane through (0, 7.5, 0) normal (0, -1, 0) x (1, 0, 0) in component "Static"
  circle A0 centre (0, 0) radius 4
  circle A1 centre (0, 0) radius 11.1
  circle A2 centre (0, 0) radius 11.1
  circle A3 centre (0, 0) radius 9.1
  dimension "d98" = -2
extrude "Extrude4" add sketch "Sketch7" along normal up to surface (0.5 mm away) contours A1 A2 bodies 3 in component "Static"
ref_plane "WorkPlane1" through (0, 0, -25) normal (0, 0, 1) x (1, 0, 0) in component "Static"
sketch "Sketch8" plane through (0, 0, -25) normal (0, 0, 1) x (1, 0, 0) in component "Static"
  circle A0 centre (0.0267, 7) radius 7
  line L0 (11, 0) -> (-11, 0)
  line L1 (25, 12) -> (-24.995, 12)
  dimension "d102" = 14
  constraint tangent A0 L0
  measures "d102" diameter of A0
extrude "Extrude5'" add sketch "Sketch8" against normal blind 75 separate body contours A0 L1 picked at (1.7607, 8.3394) makes body 4 in component "Static"
ref_plane "WorkPlane3" through (0.0267, 6, -15) normal (0, 0, 1) x (1, 0, 0) in component "Static"
sketch "Sketch9" plane through (0, 0, -15) normal (0, 0, 1) x (1, 0, 0) in component "Static"
  line L0 (-4, 12) -> (4, 12)
  line L1 (-24.995, -0.4) -> (25, -0.4)
  line L2 (-24.995, -0.4) -> (-24.995, 12)
  line L3 (25, 12) -> (-24.995, 12)
  line L4 (-20, -0.4) -> (20, -0.4)
  line L5 (20, -0.4) -> (20, 12)
  line L6 (20, 12) -> (-20, 12)
  line L7 (-20, 12) -> (-20, -0.4)
  line L8 (-20, -0.4) -> (20, 12) construction
  line L9 (20, -0.4) -> (-20, 12) construction
  line L10 (0, 1.75) -> (0, 22.5)
  point P0 (0, 5.8)
  dimension "d106" = 40
  constraint horizontal L4
  constraint perpendicular L4 L5
  constraint parallel L4 L6
  constraint parallel L5 L7
  constraint coincident L8 P0
  constraint coincident L9 P0
  constraint coincident L1 L4.start
  constraint coincident L3 L6.end
  constraint coincident P0 L10
  measures "d106" distance of L5 L7
loft "Loft2" add profiles "Sketch9" section 1 face at (1.7607, 8.3394, -25) section 2 contours L0 L1 L3 L4 L5 L6 L7 on bodies 4 bodies 3 4 in component "Static"
component "Bearing" placed x (1, 0, 0) y (0, 1, 0) z (0, 0, 1) at (0, 0, 0)
component "Rotating" placed x (1, 0, 0) y (0, 1, 0) z (0, 0, 1) at (0, 0, 0)
component "Static" placed x (1, 0, 0) y (0, 1, 0) z (0, 0, 1) at (0, 0, 0)
